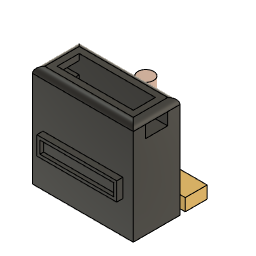
Magnetic Sliding Magnet Case v2 (Autodesk Fusion 360 design; units mm, degrees)
Autodesk Fusion 360 part; units mm, degrees
note: some values were not read from the file. Set by a fixed rule: which face or edge a step refers to.
sketch "Sketch1" plane through (0, 0, 0) normal (0, 0, 1) x (1, 0, 0)
  line L0 (28.394, 18.0448) -> (90.394, 18.0448)
  line L1 (90.394, 18.0448) -> (90.394, 36.0448)
  line L2 (90.394, 36.0448) -> (28.394, 36.0448)
  line L3 (28.394, 36.0448) -> (28.394, 18.0448)
  line L4 (100.394, 18.0448) -> (102.6874, 18.0448)
  line L5 (18.394, 46.0448) -> (102.6874, 46.0448)
  line L6 (102.6874, 46.0448) -> (102.6874, 8.0448)
  line L7 (102.6874, 8.0448) -> (18.394, 8.0448)
  line L8 (18.394, 8.0448) -> (18.394, 46.0448)
  dimension "d1" = 62
  dimension "d2" = 18
  dimension "d5" = 10
  constraint horizontal L0
  constraint vertical L1
  constraint horizontal L2
  constraint vertical L3
  constraint perpendicular L1 L4
  constraint horizontal L5
  constraint vertical L6
  constraint horizontal L7
  constraint vertical L8
  measures "d1" distance of L0.start L0.end
  measures "d2" distance of L0.start L2.end
  measures "d5" distance of L0.end L4.start
extrude "Extrude1" add sketch "Sketch1" along normal blind 10 contours L0 L1 L2 L3 makes body 1
extrude "Extrude2" add sketch "Sketch1" along normal blind 58 bodies 1
sketch "Sketch2" plane through (0, 0, 58) normal (0, 0, 1) x (-1, 0, 0)
  line L0 (-28.394, -18.0448) -> (-28.394, -36.0448)
  line L1 (-28.394, -36.0448) -> (-90.394, -36.0448)
  line L2 (-90.394, -36.0448) -> (-90.394, -18.0448)
  line L3 (-90.394, -18.0448) -> (-28.394, -18.0448)
  line L4 (-18.394, -8.0448) -> (-102.6874, -8.0448)
  line L5 (-102.6874, -8.0448) -> (-102.6874, -46.0448)
  line L6 (-102.6874, -46.0448) -> (-18.394, -46.0448)
  line L7 (-18.394, -46.0448) -> (-18.394, -8.0448)
  line L8 (-28.394, -36.0448) -> (-18.394, -36.0448)
  line L9 (-28.394, -18.0448) -> (-18.394, -18.0448)
  line L10 (-18.394, -36.0448) -> (-90.394, -36.0448)
  line L11 (-90.394, -36.0448) -> (-90.394, -18.0448)
  line L12 (-90.394, -18.0448) -> (-18.394, -18.0448)
  line L13 (-18.394, -18.0448) -> (-18.394, -36.0448)
  constraint coincident L0.end L1.start
  constraint coincident L7 L8.end
  constraint perpendicular L7 L8
  constraint coincident L0.start L3.end
  constraint coincident L7 L9.end
  constraint perpendicular L7 L9
  constraint horizontal L10
  constraint vertical L11
  constraint horizontal L12
  constraint vertical L13
  constraint coincident L2.end L3.start
extrude "Extrude3" add sketch "Sketch2" along normal blind 10 separate body contours L0 L7 L8 L9 L10 L12 L13 | L0 L1 L2 L3 L10 L11 L12 makes body 2
move_body "Move1" bodies 2 to x (1, 0, 0) y (0, 1, 0) z (0, 0, 1) at (100, 0, 0)
extrude "Extrude4" add 1 faces at (118.394, 30.0448, 61.3333) along direction (-1, 0, 0) blind 10 on bodies 2 bodies 2
sketch "Sketch3" plane through (0, 0, 58) normal (0, 0, 1) x (-1, 0, 0)
  line L0 (-28.394, -18.0448) -> (-28.394, -36.0448)
  line L1 (-28.394, -36.0448) -> (-90.394, -36.0448)
  line L2 (-90.394, -36.0448) -> (-90.394, -18.0448)
  line L3 (-90.394, -18.0448) -> (-28.394, -18.0448)
  line L4 (-18.394, -8.0448) -> (-102.6874, -8.0448)
  line L5 (-102.6874, -46.0448) -> (-18.394, -46.0448)
  line L6 (-18.394, -46.0448) -> (-18.394, -8.0448)
extrude "Extrude5" cut 1 faces at (102.6874, 33.3781, 38.6667) along direction (-1, 0, 0) blind 2.293 on bodies 1 bodies 1
sketch "Sketch4" plane through (0, 0, 58) normal (0, 0, 1) x (-1, 0, 0)
  line L0 (-100.3944, -8.0448) -> (-100.3944, -46.0448)
  line L1 (-100.3944, -46.0448) -> (-18.394, -46.0448)
  line L2 (-18.394, -46.0448) -> (-18.394, -8.0448)
  line L3 (-18.394, -8.0448) -> (-100.3944, -8.0448)
  line L4 (-28.394, -18.0448) -> (-28.394, -36.0448)
  line L5 (-28.394, -36.0448) -> (-90.394, -36.0448)
  line L6 (-90.394, -36.0448) -> (-90.394, -18.0448)
  line L7 (-90.394, -18.0448) -> (-28.394, -18.0448)
  line L8 (-28.394, -36.0448) -> (-18.394, -36.0448)
  line L9 (-28.394, -18.0448) -> (-18.394, -18.0448)
  line L10 (-90.394, -36.0448) -> (-100.3944, -36.0448)
  line L11 (-90.394, -18.0448) -> (-100.3944, -18.0448)
  constraint coincident L4.end L5.start
  constraint coincident L2 L8.end
  constraint perpendicular L2 L8
  constraint coincident L4.start L7.end
  constraint coincident L2 L9.end
  constraint perpendicular L2 L9
  constraint coincident L5.end L6.start
  constraint coincident L0 L10.end
  constraint perpendicular L0 L10
  constraint coincident L6.end L7.start
  constraint coincident L0 L11.end
  constraint perpendicular L0 L11
extrude "Extrude6" add sketch "Sketch4" along normal blind 15 contours L0 L2 L3 L7 L9 L11 | L0 L1 L2 L5 L8 L10 bodies 1
sketch "Sketch5" plane through (0, 36.0448, 0) normal (0, -1, 0) x (1, 0, 0)
  line L0 (28.394, 10) -> (90.394, 10)
  line L1 (90.394, 10) -> (90.394, 58)
  line L2 (90.394, 58) -> (100.3944, 58)
  line L3 (100.3944, 58) -> (100.3944, 73)
  line L4 (100.3944, 73) -> (18.394, 73)
  line L5 (18.394, 73) -> (18.394, 58)
  line L6 (18.394, 58) -> (28.394, 58)
  line L7 (28.394, 58) -> (28.394, 10)
  line L8 (18.394, 73) -> (28.394, 73)
  line L9 (28.394, 73) -> (28.394, 68)
  line L10 (28.394, 68) -> (18.394, 68)
  line L11 (18.394, 68) -> (18.394, 73)
  line L12 (100.3944, 73) -> (90.3944, 73)
  line L13 (90.3944, 73) -> (90.3944, 68)
  line L14 (90.3944, 68) -> (100.3944, 68)
  line L15 (100.3944, 68) -> (100.3944, 73)
  dimension "d19" = 10
  dimension "d20" = 5
  dimension "d21" = 10
  dimension "d22" = 5
  constraint horizontal L8
  constraint vertical L9
  constraint horizontal L10
  constraint vertical L11
  constraint coincident L4.end L5.start
  constraint horizontal L12
  constraint vertical L13
  constraint horizontal L14
  constraint vertical L15
  constraint coincident L3.end L4.start
  measures "d19" distance of L4.end L8.end
  measures "d20" distance of L4.end L10.end
  measures "d21" distance of L3.end L12.end
  measures "d22" distance of L3.end L14.end
extrude "Extrude7" add sketch "Sketch5" along normal blind 18 contours L4 L5 L8 L9 L10 L11 | L3 L4 L12 L13 L14 L15 bodies 1
extrude "Extrude8" cut 1 faces at (135.7274, 36.0448, 64.6667) along direction (0, -1, 0) blind 0.1 on bodies 2 bodies 2
extrude "Extrude9" cut 1 faces at (163.0607, 18.0448, 64.6667) along direction (0, 1, 0) blind 0.1 on bodies 2 bodies 2
fillet "Fillet1" radius 5 4 edges at (18.394, 27.0448, 73) (59.3942, 46.0448, 73) (100.3944, 27.0448, 73) (59.3942, 8.0448, 73) on bodies 1
sketch "Sketch6" plane through (0, 8.0448, 0) normal (0, -1, 0) x (1, 0, 0)
  line L0 (100.3944, 68) -> (18.394, 68)
  line L1 (18.394, 68) -> (18.394, 0)
  line L2 (18.394, 0) -> (100.3944, 0)
  line L3 (100.3944, 0) -> (100.3944, 68)
  line L4 (29.3942, 39) -> (89.3942, 39)
  line L5 (89.3942, 39) -> (89.3942, 29)
  line L6 (89.3942, 29) -> (29.3942, 29)
  line L7 (29.3942, 29) -> (29.3942, 39)
  line L8 (26.8942, 26.5) -> (91.8942, 26.5)
  line L9 (91.8942, 26.5) -> (91.8942, 41.5)
  line L10 (91.8942, 41.5) -> (26.8942, 41.5)
  line L11 (26.8942, 41.5) -> (26.8942, 26.5)
  dimension "d34" = 10
  constraint horizontal L4
  constraint vertical L5
  constraint horizontal L6
  constraint vertical L7
  constraint horizontal L8
  constraint vertical L9
  constraint horizontal L10
  constraint vertical L11
  measures "d34" distance of L4.start L6.end
extrude "Extrude10" add sketch "Sketch6" along normal blind 2 contours L4 L5 L6 L7 bodies 1
extrude "Extrude11" add sketch "Sketch6" along normal blind 4.5 contours L8 L9 L10 L11 bodies 1
extrude "Extrude12" add 1 faces at (49.3942, 3.5448, 27.3333) along direction (0, -1, 0) blind 0.5 on bodies 1 bodies 1
move_body "Move2" bodies 2 to x (1, 0, 0) y (0, 1, 0) z (0, 0, 1) at (0, 0, -58)
sketch "Sketch7" plane through (0, 0, 10) normal (0, 0, 1) x (-1, 0, 0)
  line L0 (-108.394, -18.1448) -> (-190.394, -18.1448)
  line L1 (-190.394, -18.1448) -> (-190.394, -35.9448)
  line L2 (-190.394, -35.9448) -> (-108.394, -35.9448)
  line L3 (-108.394, -35.9448) -> (-108.394, -18.1448)
  circle A0 centre (-128.394, -27.0448) radius 6.5
  dimension "d48" = 13
  measures "d48" diameter of A0
extrude "Extrude13" cut sketch "Sketch7" against normal blind 5 contours A0 bodies 2
sketch "Sketch8" plane through (0, 0, 0) normal (0, 0, 1) x (1, 0, 0)
  circle A0 centre (128.5884, 47.8482) radius 6.4
  dimension "d51" = 12.8
  measures "d51" diameter of A0
extrude "Extrude14" add sketch "Sketch8" along normal blind 50 separate body makes body 3
move_body "Move3" bodies 2 3 to x (1, 0, 0) y (0, 1, 0) z (0, 0, 1) at (-90.2789, 32.504, 0)
split "Split1" by plane through (0, 0, 58) normal (0, 0, 1) bodies 1 makes body 4 at (69.7275, 36.0448, 64.6667)
move_body "Move4" bodies 4 to x (1, 0, 0) y (0, 1, 0) z (0, 0, 1) at (0, 0, 10)
extrude "Extrude15" add 4 faces at (69.7275, 11.3781, 58) (93.7275, 30.0448, 58) (49.0608, 42.7115, 58) (21.7274, 30.0448, 58) along direction (0, 0, 1) blind 10 on bodies 1 bodies 1 4
